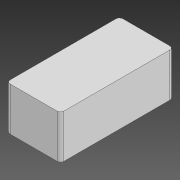
# Autodesk Inventor part: CH_01_0043_camera_PH
Saved by Autodesk Inventor 2022 (Build 260153000, 153)
## iProperties
Created: 2022-08-11
Part Number: CH_01_0043_camera_PH
Material: Generic
Document SubType Name: Modeling
Designer: Tomasz Krakowski
Density: 1 g/cm^3
Appearance: Default
Author: Tomasz Krakowski
Autodesk Inventor part; units mm, degrees
ref_plane "YZ Plane" through (0, 0, 0) normal (1, 0, 0) x (0, 1, 0)
ref_plane "XZ Plane" through (0, 0, 0) normal (0, 1, 0) x (-1, 0, 0)
ref_plane "XY Plane" through (0, 0, 0) normal (0, 0, 1) x (1, 0, 0)
sketch "Sketch1" plane through (0, 0, 0) normal (0, 1, 0) x (-1, 0, 0)
  line L0 (-20.9, 50) -> (20.9, 50)
  line L1 (23.9, 47) -> (23.9, -47)
  line L2 (20.9, -50) -> (-20.9, -50)
  line L3 (-23.9, -47) -> (-23.9, 47)
  line L4 (-23.9, 50) -> (23.9, -50) construction
  line L5 (23.9, 50) -> (-23.9, -50) construction
  arc A0 (23.9, 47) -> (20.9, 50) centre (20.9, 47) ccw
  arc A1 (20.9, -50) -> (23.9, -47) centre (20.9, -47) ccw
  arc A2 (-23.9, -47) -> (-20.9, -50) centre (-20.9, -47) ccw
  arc A3 (-20.9, 50) -> (-23.9, 47) centre (-20.9, 47) ccw
  point P0 (0, 0)
  dimension "d0" = 47.8
  dimension "d1" = 100
  dimension "d2" = 3
  constraints: 12 end point, 8 point on circle, 8 point on line, 8 tangent, 4 centre point, 3 equal radius, 2 midpoint, 2 parallel, 1 horizontal, 1 perpendicular
  measures "d0" distance between parallel lines of L3 L1
  measures "d1" distance between parallel lines of L2 L0
  measures "d2" radius of A0
extrude "Extrusion1" add sketch "Sketch1" along normal blind 38.5
body "Solid1"
